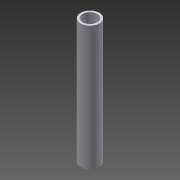
# Autodesk Inventor part: Rura_pionowa_do_kol_tylnych
Saved by Autodesk Inventor 2015 (Build 190159000, 159)
## iProperties
Created: 2015-12-01
Part Number: Rura_pionowa_do_kol_tylnych
Material: Aluminium AW-7020
Document SubType Name: Modeling
Designer: graaapsik
Density: 2.78 g/cm^3
Appearance: Aluminium AW-7020
Mass: 33.5371 g
Surface Area: 122.648 cm^2
Volume: 12.0637 cm^3
Author: graaapsik
Autodesk Inventor part; units mm, degrees
ref_plane "YZ Plane" through (0, 0, 0) normal (1, 0, 0) x (0, 1, 0)
ref_plane "XZ Plane" through (0, 0, 0) normal (0, 1, 0) x (-1, 0, 0)
ref_plane "Płaszczyzna konstrukcyjna1" through (0, 0, -16) normal (0, 0, 1) x (1, 0, 0)
sketch "Szkic1" plane through (0, 0, -16) normal (0, 0, 1) x (1, 0, 0)
  circle A0 centre (150, 0) radius 9
  point P0 (0, 0)
  dimension "d1" = 18
  dimension "d2" = 150
  constraints: 1 centre point
  measures "d1" diameter of A0
  measures "d2" distance of A0.centre point (0, 0)
extrude "Wyciągnięcie proste1" add sketch "Szkic1" against normal blind 120
shell "Skorupa2" thickness 2 removed faces 2 at (149.6384, 2.632, -16) at (149.6384, 2.632, -136)
